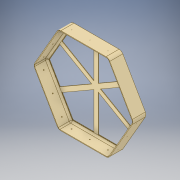
# Autodesk Inventor part: Base
Saved by Autodesk Inventor 2019 (Build 230136000, 136)
## iProperties
Created: 2021-07-14
Part Number: Base
Material: Generic
Document SubType Name: Modeling
Designer: Lix
Density: 1 g/cm^3
Appearance: Beige
Author: Lix
Autodesk Inventor part; units mm, degrees
sketch "Sketch1" plane through (0, 0, 0) normal (0, 0, 1) x (1, 0, 0)
  line L0 (57.735, -100) -> (-57.735, -100)
  line L1 (-57.735, -100) -> (-115.4701, 0)
  line L2 (-115.4701, 0) -> (-57.735, 100)
  line L3 (-57.735, 100) -> (57.735, 100)
  line L4 (57.735, 100) -> (115.4701, 0)
  line L5 (115.4701, 0) -> (57.735, -100)
  point P0 (0, 0)
  point P1 (0, 0)
  dimension "d0" = 200
  constraints: 12 end point, 1 coincident, 1 horizontal, 13 other
  measures "d0" distance between parallel lines of L5 L2
extrude "Extrusion1" add sketch "Sketch1" along normal blind 30
shell "Shell1" thickness 1.5 removed faces 1 at (19.245, 33.3333, 30) ; own thickness 1 on faces at (19.245, 33.3333, 0)
sketch "Sketch2" plane through (-113.738, 0, 30) normal (0.8660254, 0.5, 0) x (0, 0, -1)
  circle A0 centre (14.5, -98.738) radius 1
  circle A1 centre (14.5, -15) radius 1
  line L0 (29, -113.738) -> (0, -113.738) projected
  line L1 (29, 0) -> (0, 0) projected
  circle A2 centre (14.5, -56.869) radius 1
  line L2 (29, -113.738) -> (29, 0) projected
  line L3 (29, 0) -> (0, 0) projected
  line L4 (0, -113.738) -> (0, 0) projected
  line L5 (29, -113.738) -> (0, -113.738) projected
  line L6 (0, -113.738) -> (0, 0) projected
  point P0 (30, -56.869)
  point P1 (14.5, -113.738)
  point P2 (0, -56.869)
  dimension "d5" = 2
  dimension "d6" = 15
  dimension "d7" = 15
  constraints: 3 centre point, 3 vertical alignment, 2 equal radius, 2 midpoint, 1 horizontal alignment
  measures "d5" diameter of A0
  measures "d6" distance of A0.centre point (14.5, -113.738)
  measures "d7" distance from line of L1 A1.centre
ref_plane "Work Plane1" through (-28.8675, 50, 30) normal (0.8660254, 0.5, 0) x (0, 0, -1)
ref_plane "Work Plane2" through (-57.735, 0, 0) normal (0, 1, 0) x (1, 0, 0)
ref_plane "Work Plane3" through (-28.8675, -50, 0) normal (-0.8660254, 0.5, 0) x (0, 0, 1)
extrude "Extrusion2" cut sketch "Sketch2" against normal blind 1 contours A0 | A1 | A2
mirror "Mirror1" about plane through (-28.8675, 50, 30) normal (0.8660254, 0.5, 0) of "Extrusion2"
mirror "Mirror2" about plane through (-57.735, 0, 0) normal (0, 1, 0) of "Extrusion2"
mirror "Mirror3" about plane through (-28.8675, -50, 0) normal (-0.8660254, 0.5, 0) of "Extrusion2", "Mirror2"
mirror "Mirror4" about plane through (-57.735, 0, 0) normal (0, 1, 0) of "Extrusion2", "Mirror2", "Mirror3"
fillet "Fillet1" radius 4 12 edges at (0, -98.5, 1) (-85.3035, -49.25, 1) (85.3035, -49.25, 1) (85.3035, 49.25, 1) (0, 98.5, 1) (-85.3035, 49.25, 1) (-113.738, 0, 15.5) (-56.869, 98.5, 15.5) (56.869, 98.5, 15.5) (113.738, 0, 15.5) (56.869, -98.5, 15.5) (-56.869, -98.5, 15.5)
fillet "Fillet2" radius 10 6 edges at (115.4701, 0, 15) (57.735, 100, 15) (-57.735, 100, 15) (57.735, -100, 15) (-115.4701, 0, 15) (-57.735, -100, 15)
sketch "Sketch3" plane through (-56.869, -98.5, 1) normal (0, 0, 1) x (1, 0, 0)
  line L0 (61.869, 5) -> (61.869, 192) construction
  line L1 (51.869, 192) -> (51.869, 5) construction
  line L2 (51.869, 5) -> (61.869, 192) construction
  line L3 (61.869, 5) -> (51.869, 192) construction
  line L4 (-21.6044, 47.4199) -> (140.3424, 140.9199) construction
  line L5 (135.3424, 149.5801) -> (-26.6044, 56.0801) construction
  line L6 (140.3424, 56.0801) -> (-21.6044, 149.5801) construction
  line L7 (-26.6044, 140.9199) -> (135.3424, 47.4199) construction
  line L8 (-26.6044, 140.9199) -> (46.869, 98.5)
  line L9 (46.869, 98.5) -> (-26.6044, 56.0801)
  line L10 (-21.6044, 47.4199) -> (51.869, 89.8397)
  line L11 (51.869, 89.8397) -> (51.869, 5)
  line L12 (2.8868, 5) -> (-21.6044, 47.4199)
  line L13 (-26.6044, 56.0801) -> (-51.0955, 98.5)
  line L14 (110.8513, 5) -> (61.869, 5)
  line L15 (51.869, 5) -> (2.8868, 5)
  line L16 (2.8868, 192) -> (51.869, 192)
  line L17 (61.869, 192) -> (110.8513, 192)
  line L18 (110.8513, 192) -> (135.3424, 149.5801)
  line L19 (140.3424, 140.9199) -> (164.8335, 98.5)
  line L20 (164.8335, 98.5) -> (140.3424, 56.0801)
  line L21 (135.3424, 47.4199) -> (110.8513, 5)
  line L22 (61.869, 5) -> (61.869, 89.8397)
  line L23 (61.869, 89.8397) -> (135.3424, 47.4199)
  line L24 (140.3424, 56.0801) -> (66.869, 98.5)
  line L25 (66.869, 98.5) -> (140.3424, 140.9199)
  line L26 (135.3424, 149.5801) -> (61.869, 107.1603)
  line L27 (61.869, 107.1603) -> (61.869, 192)
  line L28 (2.3094, 193) -> (111.4286, 193) projected
  line L29 (51.869, 107.1603) -> (51.869, 192)
  line L30 (51.869, 107.1603) -> (-21.6044, 149.5801)
  line L31 (-51.0955, 98.5) -> (-26.6044, 140.9199)
  line L32 (-21.6044, 149.5801) -> (2.8868, 192)
  point P0 (56.869, 98.5)
  dimension "d15" = 10
  dimension "d18" = 360
  dimension "d22" = 10
  constraints: 64 end point, 11 point on line, 3 collinear, 3 perpendicular, 2 midpoint, 2 parallel, 19 other
  measures "d15" distance of L1.start L0.end
  measures "d22" distance between parallel lines of L7 L6
extrude "Extrusion3" cut sketch "Sketch3" against normal blind 10
equation "\"d7\" = d6"
body "Solid1"
